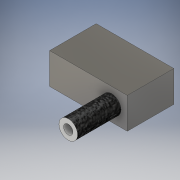
# Autodesk Inventor part: servo part
Saved by Autodesk Inventor 2019 (Build 230136000, 136)
## iProperties
Created: 2020-02-19
Part Number: servo part
Material: Generic
Document SubType Name: Modeling
Designer: LENOVO
Density: 1 g/cm^3
Appearance: Default
Author: LENOVO
Autodesk Inventor part; units mm, degrees
ref_plane "YZ Plane" through (0, 0, 0) normal (1, 0, 0) x (0, 1, 0)
ref_plane "XZ Plane" through (0, 0, 0) normal (0, 1, 0) x (-1, 0, 0)
ref_plane "XY Plane" through (0, 0, 0) normal (0, 0, 1) x (1, 0, 0)
sketch "Sketch1" plane through (0, 0, 0) normal (0, 0, 1) x (1, 0, 0)
  line L0 (0, 0) -> (25, 0)
  line L1 (25, 0) -> (25, 10)
  line L2 (25, 10) -> (0, 10)
  line L3 (0, 10) -> (0, 0)
  dimension "d0" = 25
  dimension "d1" = 10
  constraints: 8 end point, 2 parallel, 1 horizontal, 1 perpendicular
  measures "d0" distance of L2.end L1.end
  measures "d1" distance of L1.end L0.end
extrude "Extrusion1" add sketch "Sketch1" along normal blind 15
sketch "Sketch2" plane through (0, 0, 15) normal (0, 0, 1) x (1, 0, 0)
  circle A0 centre (20, 5) radius 3
  point P0 (0, 0)
  dimension "d4" = 6
  constraints: 1 centre point
  measures "d4" diameter of A0
extrude "Extrusion2" add sketch "Sketch2" along normal blind 5
sketch "Sketch3" plane through (20, 5, 20) normal (0, 0, 1) x (1, 0, 0)
  circle A0 centre (0, 0) radius 1.5
  point P0 (-20, -5)
  dimension "d7" = 3
  constraints: 1 centre point
  measures "d7" diameter of A0
extrude "Extrusion3" cut sketch "Sketch3" against normal blind 3
sketch "Sketch4" plane through (20, 5, 20) normal (0, 0, 1) x (1, 0, 0)
  circle A0 centre (0, 0) radius 3
  point P0 (-20, -5)
  constraints: 1 centre point
extrude "Extrusion4" add sketch "Sketch4" along normal blind 9
sketch "Sketch5" plane through (20, 5, 29) normal (0, 0, 1) x (1, 0, 0)
  circle A0 centre (0, 0) radius 1.5 projected
  circle A1 centre (0, 0) radius 1.5
  point P0 (-20, -5)
  constraints: 1 centre point, 1 coincident
extrude "Extrusion5" cut sketch "Sketch5" against normal blind 5
body "Solid1"
